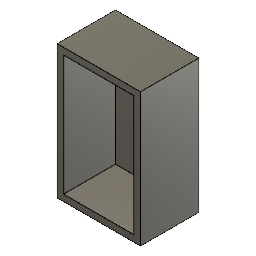
box (Autodesk Fusion 360 design; units mm, degrees)
Autodesk Fusion 360 part; units mm, degrees
box "BoxPrimitive1" add length 80 width 50 height 35 placed x (0, -1, 0) y (1, 0, 0) z (0, 0, 1) at (0, 0, 0) in component "Component"
shell "Shell1" thickness 4 removed faces 1 at (33.3333, -26.6667, 35) in component "Component"
sketch "Sketch2" plane through (0, 0, 0) normal (0, 0, 1) x (1, 0, 0) in component "Component"
component "Component" placed x (1, 0, 0) y (0, 1, 0) z (0, 0, 1) at (0, 0, 0)
